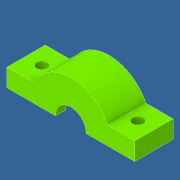
# Autodesk Inventor part: LagerKlemme
Saved by Autodesk Inventor 2016 (Build 200138000, 138)
## iProperties
Created: 2015-09-18
Part Number: LagerKlemme
Material: ABS-Kunststoff
Document SubType Name: Modeling
Designer: 4ndreas
Density: 1.06 g/cm^3
Appearance: Glatt - grün
Mass: 6.41887 g
Surface Area: 33.1193 cm^2
Volume: 6.05554 cm^3
Author: 4ndreas
Autodesk Inventor part; units mm, degrees
ref_plane "YZ Plane" through (0, 0, 0) normal (1, 0, 0) x (0, 1, 0)
ref_plane "XZ Plane" through (0, 0, 0) normal (0, 1, 0) x (-1, 0, 0)
ref_plane "XY Plane" through (0, 0, 0) normal (0, 0, 1) x (1, 0, 0)
sketch "Skizze1" plane through (0, 0, 0) normal (0, 0, 1) x (1, 0, 0)
  circle A0 centre (-18.75, 0) radius 2.1 projected
  line L0 (-6.25, 7.5) -> (-6.25, 3.5) projected
  line L1 (-6.25, 7.5) -> (-25, 7.5) projected
  line L2 (-25, 7.5) -> (-25, -7.5) projected
  line L3 (-25, -7.5) -> (-6.25, -7.5) projected
  line L4 (-6.25, -3.5) -> (-6.25, -7.5) projected
  line L5 (-11, -3.5) -> (-6.25, -3.5) projected
  line L6 (-11, 3.5) -> (-11, -3.5) projected
  line L7 (-6.25, 3.5) -> (-11, 3.5) projected
  circle A1 centre (18.75, 0) radius 2.1 projected
  line L8 (6.25, 3.5) -> (6.25, 7.5) projected
  line L9 (11, 3.5) -> (6.25, 3.5) projected
  line L10 (11, -3.5) -> (11, 3.5) projected
  line L11 (6.25, -3.5) -> (11, -3.5) projected
  line L12 (6.25, -7.5) -> (6.25, -3.5) projected
  line L13 (6.25, -7.5) -> (25, -7.5) projected
  line L14 (25, -7.5) -> (25, 7.5) projected
  line L15 (25, 7.5) -> (6.25, 7.5) projected
  line L16 (-25, 7.5) -> (25, 7.5)
  line L17 (25, 7.5) -> (25, -7.5)
  line L18 (25, -7.5) -> (-25, -7.5)
  line L19 (-25, -7.5) -> (-25, 7.5)
  line L20 (-25, 7.5) -> (25, -7.5) construction
  line L21 (25, 7.5) -> (-25, -7.5) construction
  point P0 (0, 0)
  constraints: 12 end point, 2 midpoint, 2 parallel, 1 horizontal, 1 perpendicular
extrude "Extrusion1" add sketch "Skizze1" along normal blind 16
sketch "Skizze2" plane through (-25, -7.5, 0) normal (0, -1, 0) x (1, 0, 0)
  point P0 (25, 0)
ref_plane "Arbeitsebene1" through (-25, 0, 0) normal (0, 1, 0) x (1, 0, 0)
sketch "Skizze3" plane through (-25, 0, 0) normal (0, 1, 0) x (1, 0, 0)
  line L0 (8.35, -16) -> (8.35, 0) projected
  line L1 (8.35, 0) -> (41.65, 0) projected
  line L2 (41.65, 0) -> (41.65, -16) projected
  line L3 (41.65, -16) -> (8.35, -16) projected
  line L4 (0, -16) -> (0, 0) projected
  line L5 (0, 0) -> (4.15, 0) projected
  line L6 (4.15, 0) -> (4.15, -16) projected
  line L7 (4.15, -16) -> (0, -16) projected
  line L8 (50, 0) -> (50, -16) projected
  line L9 (50, -16) -> (45.85, -16) projected
  line L10 (45.85, -16) -> (45.85, 0) projected
  line L11 (45.85, 0) -> (50, 0) projected
  circle A0 centre (25, 0) radius 11
  dimension "d2" = 22
  constraints: 1 centre point, 1 coincident
  measures "d2" diameter of A0
extrude "Extrusion2" cut sketch "Skizze3" along normal mid plane 7 contours A0 L1 | L1 A0
sketch "Skizze4" plane through (-25, 7.5, 0) normal (0, 1, 0) x (1, 0, 0)
  line L0 (50, 0) -> (50, -16) projected
  line L1 (50, -16) -> (0, -16) projected
  line L2 (0, -16) -> (0, 0) projected
  line L3 (0, 0) -> (50, 0) projected
  line L4 (50, 0) -> (50, -16) projected
  line L5 (50, -16) -> (0, -16) projected
  line L6 (0, -16) -> (0, 0) projected
  line L7 (0, 0) -> (50, 0) projected
  line L8 (50, 0) -> (50, -16) projected
  line L9 (50, -16) -> (0, -16) projected
  line L10 (0, -16) -> (0, 0) projected
  line L11 (0, 0) -> (50, 0) projected
  line L12 (50, 0) -> (50, -16) projected
  line L13 (50, -16) -> (0, -16) projected
  line L14 (0, -16) -> (0, 0) projected
  line L15 (0, 0) -> (50, 0) projected
  line L16 (14, 0) -> (36, 0) projected
  arc A0 (14, 0) -> (36, 0) centre (25, 0) ccw projected
  arc A1 (10.6125, -7) -> (39.3875, -7) centre (25, 0) ccw
  line L17 (50, -16) -> (0, -16) projected
  line L18 (39.3875, -7) -> (50, -7)
  line L19 (10.6125, -7) -> (0, -7)
  dimension "d5" = 7
  constraints: 4 end point, 2 perpendicular, 2 point on circle, 2 point on line, 1 centre point, 1 coincident, 1 collinear, 1 tangent
  measures "d5" distance between parallel lines of L3 L18
extrude "Extrusion3" cut sketch "Skizze4" against normal through all contours L0 L1 A1 L18 | L1 L2 L19 A1
sketch "Skizze5" plane through (-25, -7.5, 0) normal (0, -1, 0) x (1, 0, 0)
  circle A0 centre (25, 0) radius 6
  dimension "d8" = 12
  constraints: 1 centre point, 1 coincident
  measures "d8" diameter of A0
extrude "Extrusion4" cut sketch "Skizze5" against normal through all
